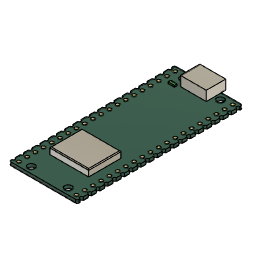
Pico W v1 (Autodesk Fusion 360 design; units mm, degrees)
Autodesk Fusion 360 part; units mm, degrees
note: some values were not read from the file. Chosen so that the rebuilt part matches the saved one: which pieces of a blend or face edit are solid.
sketch "Sketch1" plane through (0, 0, 0) normal (0, 0, 1) x (1, 0, 0)
  line L0 (0.5, 0) -> (20.5, 0)
  line L1 (21, 0.5) -> (21, 50.5)
  line L2 (20.5, 51) -> (0.5, 51)
  line L3 (0, 50.5) -> (0, 0.5)
  arc A0 (0.5, 51) -> (0, 50.5) centre (0.5, 50.5) ccw
  arc A1 (21, 50.5) -> (20.5, 51) centre (20.5, 50.5) ccw
  arc A2 (20.5, 0) -> (21, 0.5) centre (20.5, 0.5) ccw
  arc A3 (0, 0.5) -> (0.5, 0) centre (0.5, 0.5) ccw
  circle A4 centre (4.8, 49) radius 1.05
  circle A5 centre (16.2, 49) radius 1.05
  circle A6 centre (4.8, 2) radius 1.05
  circle A7 centre (16.2, 2) radius 1.05
  circle A8 centre (0, 36.93) radius 0.5
  circle A9 centre (0, 39.47) radius 0.5
  circle A10 centre (0, 42.01) radius 0.5
  circle A11 centre (0, 44.55) radius 0.5
  circle A12 centre (0, 47.09) radius 0.5
  circle A13 centre (0, 49.63) radius 0.5
  circle A14 centre (0, 34.39) radius 0.5
  circle A15 centre (0, 31.85) radius 0.5
  circle A16 centre (0, 26.77) radius 0.5
  circle A17 centre (0, 21.69) radius 0.5
  circle A18 centre (0, 24.23) radius 0.5
  circle A19 centre (0, 29.31) radius 0.5
  circle A20 centre (0, 19.15) radius 0.5
  circle A21 centre (0, 16.61) radius 0.5
  circle A22 centre (0, 11.53) radius 0.5
  circle A23 centre (0, 6.45) radius 0.5
  circle A24 centre (0, 8.99) radius 0.5
  circle A25 centre (0, 14.07) radius 0.5
  circle A26 centre (0, 3.91) radius 0.5
  circle A27 centre (0, 1.37) radius 0.5
  circle A28 centre (1.61, 24.23) radius 0.5
  circle A29 centre (1.61, 16.61) radius 0.5
  circle A30 centre (1.61, 14.07) radius 0.5
  circle A31 centre (1.61, 34.39) radius 0.5
  circle A32 centre (1.61, 47.09) radius 0.5
  circle A33 centre (1.61, 21.69) radius 0.5
  circle A34 centre (1.61, 29.31) radius 0.5
  circle A35 centre (1.61, 11.53) radius 0.5
  circle A36 centre (1.61, 6.45) radius 0.5
  circle A37 centre (1.61, 8.99) radius 0.5
  circle A38 centre (1.61, 19.15) radius 0.5
  circle A39 centre (1.61, 49.63) radius 0.5
  circle A40 centre (1.61, 31.85) radius 0.5
  circle A41 centre (1.61, 26.77) radius 0.5
  circle A42 centre (1.61, 3.91) radius 0.5
  circle A43 centre (1.61, 39.47) radius 0.5
  circle A44 centre (1.61, 42.01) radius 0.5
  circle A45 centre (1.61, 44.55) radius 0.5
  circle A46 centre (1.61, 36.93) radius 0.5
  circle A47 centre (1.61, 1.37) radius 0.5
  circle A48 centre (19.39, 8.99) radius 0.5
  circle A49 centre (19.39, 11.53) radius 0.5
  circle A50 centre (19.39, 34.39) radius 0.5
  circle A51 centre (19.39, 16.61) radius 0.5
  circle A52 centre (19.39, 21.69) radius 0.5
  circle A53 centre (19.39, 14.07) radius 0.5
  circle A54 centre (19.39, 42.01) radius 0.5
  circle A55 centre (19.39, 1.37) radius 0.5
  circle A56 centre (19.39, 26.77) radius 0.5
  circle A57 centre (19.39, 39.47) radius 0.5
  circle A58 centre (19.39, 44.55) radius 0.5
  circle A59 centre (19.39, 36.93) radius 0.5
  circle A60 centre (19.39, 47.09) radius 0.5
  circle A61 centre (19.39, 29.31) radius 0.5
  circle A62 centre (19.39, 49.63) radius 0.5
  circle A63 centre (19.39, 3.91) radius 0.5
  circle A64 centre (19.39, 31.85) radius 0.5
  circle A65 centre (19.39, 19.15) radius 0.5
  circle A66 centre (19.39, 24.23) radius 0.5
  circle A67 centre (19.39, 6.45) radius 0.5
  circle A68 centre (21, 24.23) radius 0.5
  circle A69 centre (21, 11.53) radius 0.5
  circle A70 centre (21, 44.55) radius 0.5
  circle A71 centre (21, 19.15) radius 0.5
  circle A72 centre (21, 36.93) radius 0.5
  circle A73 centre (21, 26.77) radius 0.5
  circle A74 centre (21, 3.91) radius 0.5
  circle A75 centre (21, 47.09) radius 0.5
  circle A76 centre (21, 8.99) radius 0.5
  circle A77 centre (21, 1.37) radius 0.5
  circle A78 centre (21, 34.39) radius 0.5
  circle A79 centre (21, 49.63) radius 0.5
  circle A80 centre (21, 16.61) radius 0.5
  circle A81 centre (21, 14.07) radius 0.5
  circle A82 centre (21, 6.45) radius 0.5
  circle A83 centre (21, 29.31) radius 0.5
  circle A84 centre (21, 31.85) radius 0.5
  circle A85 centre (21, 42.01) radius 0.5
  circle A86 centre (21, 39.47) radius 0.5
  circle A87 centre (21, 21.69) radius 0.5
  point P0 (21, 0)
  point P1 (0, 51)
  dimension "d1" = 21
  dimension "d2" = 51
  dimension "d3" = 0.5
  dimension "d4" = 0.5
  dimension "d5" = 0.5
  dimension "d6" = 0.5
  dimension "d8" = 2.1
  dimension "d9" = 2.1
  dimension "d10" = 11.4
  dimension "d12" = 4.8
  dimension "d13" = 4.8
  dimension "d14" = 2
  dimension "d15" = 2.1
  dimension "d16" = 2.1
  dimension "d17" = 4.8
  dimension "d18" = 11.4
  dimension "d19" = 2
  dimension "d20" = 4.8
  dimension "d21" = 1
  dimension "d22" = 1
  dimension "d23" = 1
  dimension "d24" = 1
  dimension "d25" = 1
  dimension "d26" = 1
  dimension "d27" = 1
  dimension "d28" = 1
  dimension "d29" = 1
  dimension "d30" = 1
  dimension "d31" = 1
  dimension "d32" = 1
  dimension "d33" = 1
  dimension "d34" = 1
  dimension "d35" = 1
  dimension "d36" = 1
  dimension "d37" = 1
  dimension "d38" = 1
  dimension "d39" = 1
  dimension "d40" = 1
  dimension "d48" = 2.54
  dimension "d49" = 2.54
  dimension "d50" = 2.54
  dimension "d51" = 2.54
  dimension "d52" = 2.54
  dimension "d53" = 2.54
  dimension "d54" = 2.54
  dimension "d55" = 2.54
  dimension "d56" = 2.54
  dimension "d57" = 2.54
  dimension "d58" = 2.54
  dimension "d59" = 2.54
  dimension "d60" = 2.54
  dimension "d61" = 2.54
  dimension "d62" = 2.54
  dimension "d63" = 2.54
  dimension "d64" = 2.54
  dimension "d65" = 2.54
  dimension "d66" = 2.54
  dimension "d68" = 48.26
  dimension "d69" = 1.37
  constraint horizontal L0
  constraint vertical L1
  constraint horizontal L2
  constraint vertical L3
  constraint coincident P1 L2
  constraint coincident P1 L3
  constraint tangent L2 A0
  constraint tangent L3 A0
  constraint tangent L1 A1
  constraint tangent L2 A1
  constraint coincident P0 L0
  constraint coincident P0 L1
  constraint tangent L0 A2
  constraint tangent L1 A2
  constraint coincident origin L0
  constraint coincident origin L3
  constraint tangent L0 A3
  constraint tangent L3 A3
  constraint coincident L3 A8.centre
  measures "d1" distance of origin P0
  measures "d2" distance of origin P1
  measures "d3" radius of A0
  measures "d4" radius of A1
  measures "d5" radius of A2
  measures "d6" radius of A3
  measures "d8" diameter of A4
  measures "d9" diameter of A5
  measures "d10" distance of A4.centre A5.centre
  measures "d12" distance of L3 A4.centre
  measures "d13" distance of L1 A5.centre
  measures "d14" distance of L2 A5.centre
  measures "d15" diameter of A6
  measures "d16" diameter of A7
  measures "d17" distance of L3 A6.centre
  measures "d18" distance of A6.centre A7.centre
  measures "d19" distance of L0 A7.centre
  measures "d20" distance of L1 A7.centre
  measures "d21" diameter of A8
  measures "d22" diameter of A9
  measures "d23" diameter of A10
  measures "d24" diameter of A11
  measures "d25" diameter of A12
  measures "d26" diameter of A13
  measures "d27" diameter of A17
  measures "d28" diameter of A18
  measures "d29" diameter of A16
  measures "d30" diameter of A19
  measures "d31" diameter of A15
  measures "d32" diameter of A14
  measures "d33" diameter of A23
  measures "d34" diameter of A24
  measures "d35" diameter of A22
  measures "d36" diameter of A25
  measures "d37" diameter of A21
  measures "d38" diameter of A20
  measures "d39" diameter of A26
  measures "d40" diameter of A27
  measures "d48" distance of A26.centre A27.centre
  measures "d49" distance of A23.centre A26.centre
  measures "d50" distance of A23.centre A24.centre
  measures "d51" distance of A22.centre A24.centre
  measures "d52" distance of A25.centre A22.centre
  measures "d53" distance of A25.centre A21.centre
  measures "d54" distance of A20.centre A21.centre
  measures "d55" distance of A17.centre A20.centre
  measures "d56" distance of A17.centre A18.centre
  measures "d57" distance of A16.centre A18.centre
  measures "d58" distance of A19.centre A16.centre
  measures "d59" distance of A19.centre A15.centre
  measures "d60" distance of A14.centre A15.centre
  measures "d61" distance of A8.centre A14.centre
  measures "d62" distance of A8.centre A9.centre
  measures "d63" distance of A9.centre A10.centre
  measures "d64" distance of A10.centre A11.centre
  measures "d65" distance of A11.centre A12.centre
  measures "d66" distance of A12.centre A13.centre
  measures "d68" distance of A13.centre A27.centre
  measures "d69" distance of L2 A13.centre
extrude "Extrude1" add sketch "Sketch1" along normal blind 1 contours L0 L1 L2 L3 A0 A1 A2 A3 A8 A9 A10 A11 A12 A13 A14 A15 A16 A17 A18 A19 A20 A21 A22 A23 A24 A25 A26 A27 A68 A69 A70 A71 A72 A73 A74 A75 A76 A77 A78 A79 A80 A81 A82 A83 A84 A85 A86 A87
sketch "Sketch2" plane through (0, 0, 1) normal (0, 0, 1) x (-1, 0, 0)
  circle A0 centre (-1.61, -21.69) radius 0.5
  circle A1 centre (-1.61, -47.09) radius 0.5
  circle A2 centre (-1.61, -34.39) radius 0.5
  circle A3 centre (-1.61, -14.07) radius 0.5
  circle A4 centre (-1.61, -16.61) radius 0.5
  circle A5 centre (-1.61, -24.23) radius 0.5
  circle A6 centre (-16.2, -2) radius 1.05
  circle A7 centre (-19.39, -6.45) radius 0.5
  circle A8 centre (-19.39, -24.23) radius 0.5
  circle A9 centre (-19.39, -19.15) radius 0.5
  circle A10 centre (-19.39, -31.85) radius 0.5
  circle A11 centre (-19.39, -3.91) radius 0.5
  circle A12 centre (-19.39, -49.63) radius 0.5
  circle A13 centre (-19.39, -29.31) radius 0.5
  circle A14 centre (-19.39, -47.09) radius 0.5
  circle A15 centre (-19.39, -36.93) radius 0.5
  circle A16 centre (-19.39, -44.55) radius 0.5
  circle A17 centre (-19.39, -39.47) radius 0.5
  circle A18 centre (-19.39, -26.77) radius 0.5
  circle A19 centre (-19.39, -1.37) radius 0.5
  circle A20 centre (-19.39, -42.01) radius 0.5
  circle A21 centre (-19.39, -14.07) radius 0.5
  circle A22 centre (-19.39, -21.69) radius 0.5
  circle A23 centre (-19.39, -16.61) radius 0.5
  circle A24 centre (-19.39, -34.39) radius 0.5
  circle A25 centre (-19.39, -11.53) radius 0.5
  circle A26 centre (-19.39, -8.99) radius 0.5
  circle A27 centre (-1.61, -1.37) radius 0.5
  circle A28 centre (-1.61, -29.31) radius 0.5
  circle A29 centre (-1.61, -11.53) radius 0.5
  circle A30 centre (-1.61, -6.45) radius 0.5
  circle A31 centre (-4.8, -2) radius 1.05
  circle A32 centre (-16.2, -49) radius 1.05
  circle A33 centre (-4.8, -49) radius 1.05
  circle A34 centre (-1.61, -8.99) radius 0.5
  circle A35 centre (-1.61, -19.15) radius 0.5
  circle A36 centre (-1.61, -49.63) radius 0.5
  circle A37 centre (-1.61, -44.55) radius 0.5
  circle A38 centre (-1.61, -36.93) radius 0.5
  circle A39 centre (-1.61, -42.01) radius 0.5
  circle A40 centre (-1.61, -39.47) radius 0.5
  circle A41 centre (-1.61, -3.91) radius 0.5
  circle A42 centre (-1.61, -26.77) radius 0.5
  circle A43 centre (-1.61, -31.85) radius 0.5
  line L0 (-21, -17.11) -> (-21, -18.65)
  arc A44 (-21, -19.65) -> (-21, -18.65) centre (-21, -19.15) ccw
  line L1 (-21, -19.65) -> (-21, -21.19)
  arc A45 (-21, -22.19) -> (-21, -21.19) centre (-21, -21.69) ccw
  line L2 (-21, -22.19) -> (-21, -23.73)
  arc A46 (-21, -24.73) -> (-21, -23.73) centre (-21, -24.23) ccw
  line L3 (-21, -24.73) -> (-21, -26.27)
  arc A47 (-21, -27.27) -> (-21, -26.27) centre (-21, -26.77) ccw
  line L4 (-21, -27.27) -> (-21, -28.81)
  arc A48 (-21, -29.81) -> (-21, -28.81) centre (-21, -29.31) ccw
  line L5 (-21, -29.81) -> (-21, -31.35)
  arc A49 (-21, -32.35) -> (-21, -31.35) centre (-21, -31.85) ccw
  line L6 (-21, -32.35) -> (-21, -33.89)
  arc A50 (-21, -34.89) -> (-21, -33.89) centre (-21, -34.39) ccw
  line L7 (-21, -34.89) -> (-21, -36.43)
  arc A51 (-21, -37.43) -> (-21, -36.43) centre (-21, -36.93) ccw
  line L8 (-21, -37.43) -> (-21, -38.97)
  arc A52 (-21, -39.97) -> (-21, -38.97) centre (-21, -39.47) ccw
  line L9 (-21, -39.97) -> (-21, -41.51)
  arc A53 (-21, -42.51) -> (-21, -41.51) centre (-21, -42.01) ccw
  line L10 (-21, -42.51) -> (-21, -44.05)
  arc A54 (-21, -45.05) -> (-21, -44.05) centre (-21, -44.55) ccw
  line L11 (-21, -45.05) -> (-21, -46.59)
  arc A55 (-21, -47.59) -> (-21, -46.59) centre (-21, -47.09) ccw
  line L12 (-21, -47.59) -> (-21, -49.13)
  arc A56 (-21, -50.13) -> (-21, -49.13) centre (-21, -49.63) ccw
  line L13 (-21, -50.13) -> (-21, -50.5)
  arc A57 (-21, -50.5) -> (-20.5, -51) centre (-20.5, -50.5) ccw
  line L14 (-20.5, -51) -> (-0.5, -51)
  arc A58 (-0.5, -51) -> (0, -50.5) centre (-0.5, -50.5) ccw
  line L15 (0, -50.5) -> (0, -50.13)
  arc A59 (0, -49.13) -> (0, -50.13) centre (0, -49.63) ccw
  line L16 (0, -49.13) -> (0, -47.59)
  arc A60 (0, -46.59) -> (0, -47.59) centre (0, -47.09) ccw
  line L17 (0, -46.59) -> (0, -45.05)
  arc A61 (0, -44.05) -> (0, -45.05) centre (0, -44.55) ccw
  line L18 (0, -44.05) -> (0, -42.51)
  arc A62 (0, -41.51) -> (0, -42.51) centre (0, -42.01) ccw
  line L19 (0, -41.51) -> (0, -39.97)
  arc A63 (0, -38.97) -> (0, -39.97) centre (0, -39.47) ccw
  line L20 (0, -38.97) -> (0, -37.43)
  arc A64 (0, -36.43) -> (0, -37.43) centre (0, -36.93) ccw
  line L21 (0, -36.43) -> (0, -34.89)
  arc A65 (0, -33.89) -> (0, -34.89) centre (0, -34.39) ccw
  line L22 (0, -33.89) -> (0, -32.35)
  arc A66 (0, -31.35) -> (0, -32.35) centre (0, -31.85) ccw
  line L23 (0, -31.35) -> (0, -29.81)
  arc A67 (0, -28.81) -> (0, -29.81) centre (0, -29.31) ccw
  line L24 (0, -28.81) -> (0, -27.27)
  arc A68 (0, -26.27) -> (0, -27.27) centre (0, -26.77) ccw
  line L25 (0, -26.27) -> (0, -24.73)
  arc A69 (0, -23.73) -> (0, -24.73) centre (0, -24.23) ccw
  line L26 (0, -23.73) -> (0, -22.19)
  arc A70 (0, -21.19) -> (0, -22.19) centre (0, -21.69) ccw
  line L27 (0, -21.19) -> (0, -19.65)
  arc A71 (0, -18.65) -> (0, -19.65) centre (0, -19.15) ccw
  line L28 (0, -18.65) -> (0, -17.11)
  arc A72 (0, -16.11) -> (0, -17.11) centre (0, -16.61) ccw
  line L29 (0, -16.11) -> (0, -14.57)
  arc A73 (0, -13.57) -> (0, -14.57) centre (0, -14.07) ccw
  line L30 (0, -13.57) -> (0, -12.03)
  arc A74 (0, -11.03) -> (0, -12.03) centre (0, -11.53) ccw
  line L31 (0, -11.03) -> (0, -9.49)
  arc A75 (0, -8.49) -> (0, -9.49) centre (0, -8.99) ccw
  line L32 (0, -8.49) -> (0, -6.95)
  arc A76 (0, -5.95) -> (0, -6.95) centre (0, -6.45) ccw
  line L33 (0, -5.95) -> (0, -4.41)
  arc A77 (0, -3.41) -> (0, -4.41) centre (0, -3.91) ccw
  line L34 (0, -3.41) -> (0, -1.87)
  arc A78 (0, -0.87) -> (0, -1.87) centre (0, -1.37) ccw
  line L35 (0, -0.87) -> (0, -0.5)
  arc A79 (0, -0.5) -> (-0.5, 0) centre (-0.5, -0.5) ccw
  line L36 (-0.5, 0) -> (-20.5, 0)
  arc A80 (-20.5, 0) -> (-21, -0.5) centre (-20.5, -0.5) ccw
  line L37 (-21, -0.5) -> (-21, -0.87)
  arc A81 (-21, -1.87) -> (-21, -0.87) centre (-21, -1.37) ccw
  line L38 (-21, -1.87) -> (-21, -3.41)
  arc A82 (-21, -4.41) -> (-21, -3.41) centre (-21, -3.91) ccw
  line L39 (-21, -4.41) -> (-21, -5.95)
  arc A83 (-21, -6.95) -> (-21, -5.95) centre (-21, -6.45) ccw
  line L40 (-21, -6.95) -> (-21, -8.49)
  arc A84 (-21, -9.49) -> (-21, -8.49) centre (-21, -8.99) ccw
  line L41 (-21, -9.49) -> (-21, -11.03)
  arc A85 (-21, -12.03) -> (-21, -11.03) centre (-21, -11.53) ccw
  line L42 (-21, -12.03) -> (-21, -13.57)
  arc A86 (-21, -14.57) -> (-21, -13.57) centre (-21, -14.07) ccw
  line L43 (-21, -14.57) -> (-21, -16.11)
  arc A87 (-21, -17.11) -> (-21, -16.11) centre (-21, -16.61) ccw
  line L44 (-6.5, -52.3) -> (-14.5, -52.3)
  line L45 (-14.5, -52.3) -> (-14.5, -46.3)
  line L46 (-14.5, -46.3) -> (-6.5, -46.3)
  line L47 (-6.5, -46.3) -> (-6.5, -52.3)
  dimension "d112" = 8
  dimension "d113" = 6
  dimension "d114" = 1.3
  dimension "d115" = 6.5
  constraint horizontal L44
  constraint vertical L45
  constraint horizontal L46
  constraint vertical L47
  measures "d112" distance of L44.start L44.end
  measures "d113" distance of L44.start L46.end
  measures "d114" distance of L14 L44
  measures "d115" distance of L16 L47
extrude "Extrude2" add sketch "Sketch2" along normal blind 3 contours L14 L45 L46 L47 | L14 L44 L45 L47
sketch "Sketch3" plane through (0, 0, 1) normal (0, 0, 1) x (-1, 0, 0)
  line L0 (-6.5, -46.3) -> (-6.5, -51)
  line L1 (-6.5, -51) -> (-0.5, -51)
  arc A0 (-0.5, -51) -> (0, -50.5) centre (-0.5, -50.5) ccw
  line L2 (0, -50.5) -> (0, -50.13)
  arc A1 (0, -49.13) -> (0, -50.13) centre (0, -49.63) ccw
  line L3 (0, -49.13) -> (0, -47.59)
  arc A2 (0, -46.59) -> (0, -47.59) centre (0, -47.09) ccw
  line L4 (0, -46.59) -> (0, -45.05)
  arc A3 (0, -44.05) -> (0, -45.05) centre (0, -44.55) ccw
  line L5 (0, -44.05) -> (0, -42.51)
  arc A4 (0, -41.51) -> (0, -42.51) centre (0, -42.01) ccw
  line L6 (0, -41.51) -> (0, -39.97)
  arc A5 (0, -38.97) -> (0, -39.97) centre (0, -39.47) ccw
  line L7 (0, -38.97) -> (0, -37.43)
  arc A6 (0, -36.43) -> (0, -37.43) centre (0, -36.93) ccw
  line L8 (0, -36.43) -> (0, -34.89)
  arc A7 (0, -33.89) -> (0, -34.89) centre (0, -34.39) ccw
  line L9 (0, -33.89) -> (0, -32.35)
  arc A8 (0, -31.35) -> (0, -32.35) centre (0, -31.85) ccw
  line L10 (0, -31.35) -> (0, -29.81)
  arc A9 (0, -28.81) -> (0, -29.81) centre (0, -29.31) ccw
  line L11 (0, -28.81) -> (0, -27.27)
  arc A10 (0, -26.27) -> (0, -27.27) centre (0, -26.77) ccw
  line L12 (0, -26.27) -> (0, -24.73)
  arc A11 (0, -23.73) -> (0, -24.73) centre (0, -24.23) ccw
  line L13 (0, -23.73) -> (0, -22.19)
  arc A12 (0, -21.19) -> (0, -22.19) centre (0, -21.69) ccw
  line L14 (0, -21.19) -> (0, -19.65)
  arc A13 (0, -18.65) -> (0, -19.65) centre (0, -19.15) ccw
  line L15 (0, -18.65) -> (0, -17.11)
  arc A14 (0, -16.11) -> (0, -17.11) centre (0, -16.61) ccw
  line L16 (0, -16.11) -> (0, -14.57)
  arc A15 (0, -13.57) -> (0, -14.57) centre (0, -14.07) ccw
  line L17 (0, -13.57) -> (0, -12.03)
  arc A16 (0, -11.03) -> (0, -12.03) centre (0, -11.53) ccw
  line L18 (0, -11.03) -> (0, -9.49)
  arc A17 (0, -8.49) -> (0, -9.49) centre (0, -8.99) ccw
  line L19 (0, -8.49) -> (0, -6.95)
  arc A18 (0, -5.95) -> (0, -6.95) centre (0, -6.45) ccw
  line L20 (0, -5.95) -> (0, -4.41)
  arc A19 (0, -3.41) -> (0, -4.41) centre (0, -3.91) ccw
  line L21 (0, -3.41) -> (0, -1.87)
  arc A20 (0, -0.87) -> (0, -1.87) centre (0, -1.37) ccw
  line L22 (0, -0.87) -> (0, -0.5)
  arc A21 (0, -0.5) -> (-0.5, 0) centre (-0.5, -0.5) ccw
  line L23 (-0.5, 0) -> (-20.5, 0)
  arc A22 (-20.5, 0) -> (-21, -0.5) centre (-20.5, -0.5) ccw
  line L24 (-21, -0.5) -> (-21, -0.87)
  arc A23 (-21, -1.87) -> (-21, -0.87) centre (-21, -1.37) ccw
  line L25 (-21, -1.87) -> (-21, -3.41)
  arc A24 (-21, -4.41) -> (-21, -3.41) centre (-21, -3.91) ccw
  line L26 (-21, -4.41) -> (-21, -5.95)
  arc A25 (-21, -6.95) -> (-21, -5.95) centre (-21, -6.45) ccw
  line L27 (-21, -6.95) -> (-21, -8.49)
  arc A26 (-21, -9.49) -> (-21, -8.49) centre (-21, -8.99) ccw
  line L28 (-21, -9.49) -> (-21, -11.03)
  arc A27 (-21, -12.03) -> (-21, -11.03) centre (-21, -11.53) ccw
  line L29 (-21, -12.03) -> (-21, -13.57)
  arc A28 (-21, -14.57) -> (-21, -13.57) centre (-21, -14.07) ccw
  line L30 (-21, -14.57) -> (-21, -16.11)
  arc A29 (-21, -17.11) -> (-21, -16.11) centre (-21, -16.61) ccw
  line L31 (-21, -17.11) -> (-21, -18.65)
  arc A30 (-21, -19.65) -> (-21, -18.65) centre (-21, -19.15) ccw
  line L32 (-21, -19.65) -> (-21, -21.19)
  arc A31 (-21, -22.19) -> (-21, -21.19) centre (-21, -21.69) ccw
  line L33 (-21, -22.19) -> (-21, -23.73)
  arc A32 (-21, -24.73) -> (-21, -23.73) centre (-21, -24.23) ccw
  line L34 (-21, -24.73) -> (-21, -26.27)
  arc A33 (-21, -27.27) -> (-21, -26.27) centre (-21, -26.77) ccw
  line L35 (-21, -27.27) -> (-21, -28.81)
  arc A34 (-21, -29.81) -> (-21, -28.81) centre (-21, -29.31) ccw
  line L36 (-21, -29.81) -> (-21, -31.35)
  arc A35 (-21, -32.35) -> (-21, -31.35) centre (-21, -31.85) ccw
  line L37 (-21, -32.35) -> (-21, -33.89)
  arc A36 (-21, -34.89) -> (-21, -33.89) centre (-21, -34.39) ccw
  line L38 (-21, -34.89) -> (-21, -36.43)
  arc A37 (-21, -37.43) -> (-21, -36.43) centre (-21, -36.93) ccw
  line L39 (-21, -37.43) -> (-21, -38.97)
  arc A38 (-21, -39.97) -> (-21, -38.97) centre (-21, -39.47) ccw
  line L40 (-21, -39.97) -> (-21, -41.51)
  arc A39 (-21, -42.51) -> (-21, -41.51) centre (-21, -42.01) ccw
  line L41 (-21, -42.51) -> (-21, -44.05)
  arc A40 (-21, -45.05) -> (-21, -44.05) centre (-21, -44.55) ccw
  line L42 (-21, -45.05) -> (-21, -46.59)
  arc A41 (-21, -47.59) -> (-21, -46.59) centre (-21, -47.09) ccw
  line L43 (-21, -47.59) -> (-21, -49.13)
  arc A42 (-21, -50.13) -> (-21, -49.13) centre (-21, -49.63) ccw
  line L44 (-21, -50.13) -> (-21, -50.5)
  arc A43 (-21, -50.5) -> (-20.5, -51) centre (-20.5, -50.5) ccw
  line L45 (-20.5, -51) -> (-14.5, -51)
  line L46 (-14.5, -51) -> (-14.5, -46.3)
  line L47 (-14.5, -46.3) -> (-6.5, -46.3)
  circle A44 centre (-1.61, -21.69) radius 0.5
  circle A45 centre (-1.61, -47.09) radius 0.5
  circle A46 centre (-1.61, -34.39) radius 0.5
  circle A47 centre (-1.61, -14.07) radius 0.5
  circle A48 centre (-1.61, -16.61) radius 0.5
  circle A49 centre (-1.61, -24.23) radius 0.5
  circle A50 centre (-16.2, -2) radius 1.05
  circle A51 centre (-19.39, -6.45) radius 0.5
  circle A52 centre (-19.39, -24.23) radius 0.5
  circle A53 centre (-19.39, -19.15) radius 0.5
  circle A54 centre (-19.39, -31.85) radius 0.5
  circle A55 centre (-19.39, -3.91) radius 0.5
  circle A56 centre (-19.39, -49.63) radius 0.5
  circle A57 centre (-19.39, -29.31) radius 0.5
  circle A58 centre (-19.39, -47.09) radius 0.5
  circle A59 centre (-19.39, -36.93) radius 0.5
  circle A60 centre (-19.39, -44.55) radius 0.5
  circle A61 centre (-19.39, -39.47) radius 0.5
  circle A62 centre (-19.39, -26.77) radius 0.5
  circle A63 centre (-19.39, -1.37) radius 0.5
  circle A64 centre (-19.39, -42.01) radius 0.5
  circle A65 centre (-19.39, -14.07) radius 0.5
  circle A66 centre (-19.39, -21.69) radius 0.5
  circle A67 centre (-19.39, -16.61) radius 0.5
  circle A68 centre (-19.39, -34.39) radius 0.5
  circle A69 centre (-19.39, -11.53) radius 0.5
  circle A70 centre (-19.39, -8.99) radius 0.5
  circle A71 centre (-1.61, -1.37) radius 0.5
  circle A72 centre (-1.61, -29.31) radius 0.5
  circle A73 centre (-1.61, -11.53) radius 0.5
  circle A74 centre (-1.61, -6.45) radius 0.5
  circle A75 centre (-4.8, -2) radius 1.05
  circle A76 centre (-16.2, -49) radius 1.05
  circle A77 centre (-4.8, -49) radius 1.05
  circle A78 centre (-1.61, -8.99) radius 0.5
  circle A79 centre (-1.61, -19.15) radius 0.5
  circle A80 centre (-1.61, -49.63) radius 0.5
  circle A81 centre (-1.61, -44.55) radius 0.5
  circle A82 centre (-1.61, -36.93) radius 0.5
  circle A83 centre (-1.61, -42.01) radius 0.5
  circle A84 centre (-1.61, -39.47) radius 0.5
  circle A85 centre (-1.61, -3.91) radius 0.5
  circle A86 centre (-1.61, -26.77) radius 0.5
  circle A87 centre (-1.61, -31.85) radius 0.5
  line L48 (-4.5, -18) -> (-16.5, -18)
  line L49 (-16.5, -18) -> (-16.5, -8)
  line L50 (-16.5, -8) -> (-4.5, -8)
  line L51 (-4.5, -8) -> (-4.5, -18)
  dimension "d118" = 12
  dimension "d119" = 10
  dimension "d120" = 4.5
  dimension "d121" = 8
  constraint horizontal L48
  constraint vertical L49
  constraint horizontal L50
  constraint vertical L51
  measures "d118" distance of L48.start L48.end
  measures "d119" distance of L48.start L50.end
  measures "d120" distance of L15 L51
  measures "d121" distance of L23 L50
extrude "Extrude3" add sketch "Sketch3" along normal blind 2 contours L48 L49 L50 L51
fillet "Fillet1" radius 0.25 4 edges at (10.5, 18, 3) (16.5, 13, 3) (10.5, 8, 3) (4.5, 13, 3)
sketch "Sketch4" plane through (0, 0, 1) normal (0, 0, 1) x (-1, 0, 0)
  line L0 (-4.5, -8) -> (-4.5, -18)
  line L1 (-4.5, -18) -> (-16.5, -18)
  line L2 (-16.5, -18) -> (-16.5, -8)
  line L3 (-16.5, -8) -> (-4.5, -8)
  line L4 (-6.5, -46.3) -> (-6.5, -51)
  line L5 (-6.5, -51) -> (-0.5, -51)
  arc A0 (-0.5, -51) -> (0, -50.5) centre (-0.5, -50.5) ccw
  line L6 (0, -50.5) -> (0, -50.13)
  arc A1 (0, -49.13) -> (0, -50.13) centre (0, -49.63) ccw
  line L7 (0, -49.13) -> (0, -47.59)
  arc A2 (0, -46.59) -> (0, -47.59) centre (0, -47.09) ccw
  line L8 (0, -46.59) -> (0, -45.05)
  arc A3 (0, -44.05) -> (0, -45.05) centre (0, -44.55) ccw
  line L9 (0, -44.05) -> (0, -42.51)
  arc A4 (0, -41.51) -> (0, -42.51) centre (0, -42.01) ccw
  line L10 (0, -41.51) -> (0, -39.97)
  arc A5 (0, -38.97) -> (0, -39.97) centre (0, -39.47) ccw
  line L11 (0, -38.97) -> (0, -37.43)
  arc A6 (0, -36.43) -> (0, -37.43) centre (0, -36.93) ccw
  line L12 (0, -36.43) -> (0, -34.89)
  arc A7 (0, -33.89) -> (0, -34.89) centre (0, -34.39) ccw
  line L13 (0, -33.89) -> (0, -32.35)
  arc A8 (0, -31.35) -> (0, -32.35) centre (0, -31.85) ccw
  line L14 (0, -31.35) -> (0, -29.81)
  arc A9 (0, -28.81) -> (0, -29.81) centre (0, -29.31) ccw
  line L15 (0, -28.81) -> (0, -27.27)
  arc A10 (0, -26.27) -> (0, -27.27) centre (0, -26.77) ccw
  line L16 (0, -26.27) -> (0, -24.73)
  arc A11 (0, -23.73) -> (0, -24.73) centre (0, -24.23) ccw
  line L17 (0, -23.73) -> (0, -22.19)
  arc A12 (0, -21.19) -> (0, -22.19) centre (0, -21.69) ccw
  line L18 (0, -21.19) -> (0, -19.65)
  arc A13 (0, -18.65) -> (0, -19.65) centre (0, -19.15) ccw
  line L19 (0, -18.65) -> (0, -17.11)
  arc A14 (0, -16.11) -> (0, -17.11) centre (0, -16.61) ccw
  line L20 (0, -16.11) -> (0, -14.57)
  arc A15 (0, -13.57) -> (0, -14.57) centre (0, -14.07) ccw
  line L21 (0, -13.57) -> (0, -12.03)
  arc A16 (0, -11.03) -> (0, -12.03) centre (0, -11.53) ccw
  line L22 (0, -11.03) -> (0, -9.49)
  arc A17 (0, -8.49) -> (0, -9.49) centre (0, -8.99) ccw
  line L23 (0, -8.49) -> (0, -6.95)
  arc A18 (0, -5.95) -> (0, -6.95) centre (0, -6.45) ccw
  line L24 (0, -5.95) -> (0, -4.41)
  arc A19 (0, -3.41) -> (0, -4.41) centre (0, -3.91) ccw
  line L25 (0, -3.41) -> (0, -1.87)
  arc A20 (0, -0.87) -> (0, -1.87) centre (0, -1.37) ccw
  line L26 (0, -0.87) -> (0, -0.5)
  arc A21 (0, -0.5) -> (-0.5, 0) centre (-0.5, -0.5) ccw
  line L27 (-0.5, 0) -> (-20.5, 0)
  arc A22 (-20.5, 0) -> (-21, -0.5) centre (-20.5, -0.5) ccw
  line L28 (-21, -0.5) -> (-21, -0.87)
  arc A23 (-21, -1.87) -> (-21, -0.87) centre (-21, -1.37) ccw
  line L29 (-21, -1.87) -> (-21, -3.41)
  arc A24 (-21, -4.41) -> (-21, -3.41) centre (-21, -3.91) ccw
  line L30 (-21, -4.41) -> (-21, -5.95)
  arc A25 (-21, -6.95) -> (-21, -5.95) centre (-21, -6.45) ccw
  line L31 (-21, -6.95) -> (-21, -8.49)
  arc A26 (-21, -9.49) -> (-21, -8.49) centre (-21, -8.99) ccw
  line L32 (-21, -9.49) -> (-21, -11.03)
  arc A27 (-21, -12.03) -> (-21, -11.03) centre (-21, -11.53) ccw
  line L33 (-21, -12.03) -> (-21, -13.57)
  arc A28 (-21, -14.57) -> (-21, -13.57) centre (-21, -14.07) ccw
  line L34 (-21, -14.57) -> (-21, -16.11)
  arc A29 (-21, -17.11) -> (-21, -16.11) centre (-21, -16.61) ccw
  line L35 (-21, -17.11) -> (-21, -18.65)
  arc A30 (-21, -19.65) -> (-21, -18.65) centre (-21, -19.15) ccw
  line L36 (-21, -19.65) -> (-21, -21.19)
  arc A31 (-21, -22.19) -> (-21, -21.19) centre (-21, -21.69) ccw
  line L37 (-21, -22.19) -> (-21, -23.73)
  arc A32 (-21, -24.73) -> (-21, -23.73) centre (-21, -24.23) ccw
  line L38 (-21, -24.73) -> (-21, -26.27)
  arc A33 (-21, -27.27) -> (-21, -26.27) centre (-21, -26.77) ccw
  line L39 (-21, -27.27) -> (-21, -28.81)
  arc A34 (-21, -29.81) -> (-21, -28.81) centre (-21, -29.31) ccw
  line L40 (-21, -29.81) -> (-21, -31.35)
  arc A35 (-21, -32.35) -> (-21, -31.35) centre (-21, -31.85) ccw
  line L41 (-21, -32.35) -> (-21, -33.89)
  arc A36 (-21, -34.89) -> (-21, -33.89) centre (-21, -34.39) ccw
  line L42 (-21, -34.89) -> (-21, -36.43)
  arc A37 (-21, -37.43) -> (-21, -36.43) centre (-21, -36.93) ccw
  line L43 (-21, -37.43) -> (-21, -38.97)
  arc A38 (-21, -39.97) -> (-21, -38.97) centre (-21, -39.47) ccw
  line L44 (-21, -39.97) -> (-21, -41.51)
  arc A39 (-21, -42.51) -> (-21, -41.51) centre (-21, -42.01) ccw
  line L45 (-21, -42.51) -> (-21, -44.05)
  arc A40 (-21, -45.05) -> (-21, -44.05) centre (-21, -44.55) ccw
  line L46 (-21, -45.05) -> (-21, -46.59)
  arc A41 (-21, -47.59) -> (-21, -46.59) centre (-21, -47.09) ccw
  line L47 (-21, -47.59) -> (-21, -49.13)
  arc A42 (-21, -50.13) -> (-21, -49.13) centre (-21, -49.63) ccw
  line L48 (-21, -50.13) -> (-21, -50.5)
  arc A43 (-21, -50.5) -> (-20.5, -51) centre (-20.5, -50.5) ccw
  line L49 (-20.5, -51) -> (-14.5, -51)
  line L50 (-14.5, -51) -> (-14.5, -46.3)
  line L51 (-14.5, -46.3) -> (-6.5, -46.3)
  circle A44 centre (-1.61, -21.69) radius 0.5
  circle A45 centre (-1.61, -47.09) radius 0.5
  circle A46 centre (-1.61, -34.39) radius 0.5
  circle A47 centre (-1.61, -14.07) radius 0.5
  circle A48 centre (-1.61, -16.61) radius 0.5
  circle A49 centre (-1.61, -24.23) radius 0.5
  circle A50 centre (-16.2, -2) radius 1.05
  circle A51 centre (-19.39, -6.45) radius 0.5
  circle A52 centre (-19.39, -24.23) radius 0.5
  circle A53 centre (-19.39, -19.15) radius 0.5
  circle A54 centre (-19.39, -31.85) radius 0.5
  circle A55 centre (-19.39, -3.91) radius 0.5
  circle A56 centre (-19.39, -49.63) radius 0.5
  circle A57 centre (-19.39, -29.31) radius 0.5
  circle A58 centre (-19.39, -47.09) radius 0.5
  circle A59 centre (-19.39, -36.93) radius 0.5
  circle A60 centre (-19.39, -44.55) radius 0.5
  circle A61 centre (-19.39, -39.47) radius 0.5
  circle A62 centre (-19.39, -26.77) radius 0.5
  circle A63 centre (-19.39, -1.37) radius 0.5
  circle A64 centre (-19.39, -42.01) radius 0.5
  circle A65 centre (-19.39, -14.07) radius 0.5
  circle A66 centre (-19.39, -21.69) radius 0.5
  circle A67 centre (-19.39, -16.61) radius 0.5
  circle A68 centre (-19.39, -34.39) radius 0.5
  circle A69 centre (-19.39, -11.53) radius 0.5
  circle A70 centre (-19.39, -8.99) radius 0.5
  circle A71 centre (-1.61, -1.37) radius 0.5
  circle A72 centre (-1.61, -29.31) radius 0.5
  circle A73 centre (-1.61, -11.53) radius 0.5
  circle A74 centre (-1.61, -6.45) radius 0.5
  circle A75 centre (-4.8, -2) radius 1.05
  circle A76 centre (-16.2, -49) radius 1.05
  circle A77 centre (-4.8, -49) radius 1.05
  circle A78 centre (-1.61, -8.99) radius 0.5
  circle A79 centre (-1.61, -19.15) radius 0.5
  circle A80 centre (-1.61, -49.63) radius 0.5
  circle A81 centre (-1.61, -44.55) radius 0.5
  circle A82 centre (-1.61, -36.93) radius 0.5
  circle A83 centre (-1.61, -42.01) radius 0.5
  circle A84 centre (-1.61, -39.47) radius 0.5
  circle A85 centre (-1.61, -3.91) radius 0.5
  circle A86 centre (-1.61, -26.77) radius 0.5
  circle A87 centre (-1.61, -31.85) radius 0.5
  line L52 (-3.8, -46) -> (-5.8, -46)
  line L53 (-5.8, -46) -> (-5.8, -45.2)
  line L54 (-5.8, -45.2) -> (-3.8, -45.2)
  line L55 (-3.8, -45.2) -> (-3.8, -46)
  dimension "d126" = 2
  dimension "d127" = 0.8
  dimension "d128" = 5
  dimension "d129" = 3.8
  constraint horizontal L52
  constraint vertical L53
  constraint horizontal L54
  constraint vertical L55
  measures "d126" distance of L52.start L52.end
  measures "d127" distance of L52.start L54.end
  measures "d128" distance of L5 L52
  measures "d129" distance of L7 L55
extrude "Extrude4" add sketch "Sketch4" along normal blind 0.5 contours L52 L53 L54 L55
move_body "Move1" bodies 1 to x (1, 0, 0) y (0, 1, 0) z (0, 0, 1) at (0, 0, 9)
sketch "Sketch6" plane through (0, 0, 0) normal (0, 0, 1) x (1, 0, 0)
shell "Shell1" thickness 0.2 removed faces 1 at (9.1667, 52.3, 11)
